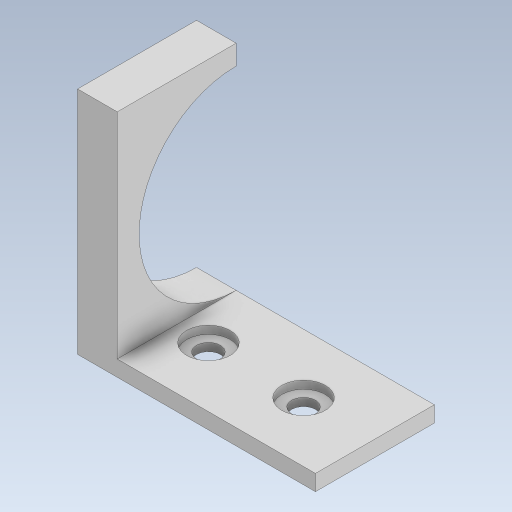
# Autodesk Inventor part: Bracket Motor JGA Kiri
Saved by Autodesk Inventor 2023.5 (Build 275446000, 446)
## iProperties
Created: 2025-09-12
Part Number: Bracket Motor JGA Kiri
Material: Generic
Document SubType Name: Modeling
Designer: Guntur
Density: 1 g/cm^3
Appearance: Default
Author: Guntur
## iProperties of the stored document Bracket Motor JGA Kiri_3DPrint.ipt
Created: 2025-09-14
Part Number: Bracket Motor JGA Kiri_3DPrint
Material: Generic
Document SubType Name: Modeling
Designer: Guntur
Density: 1 g/cm^3
Appearance: Default
Author: Guntur
Autodesk Inventor part; units mm, degrees
ref_plane "YZ Plane" through (0, 0, 0) normal (1, 0, 0) x (0, 1, 0)
ref_plane "XZ Plane" through (0, 0, 0) normal (0, 1, 0) x (-1, 0, 0)
ref_plane "XY Plane" through (0, 0, 0) normal (0, 0, 1) x (1, 0, 0)
sketch "Sketch1" plane through (0, 0, 0) normal (0, 1, 0) x (-1, 0, 0)
  line L0 (15, 7.5) -> (-15, 7.5)
  line L1 (-15, 7.5) -> (-15, -7.5)
  line L2 (-15, -7.5) -> (15, -7.5)
  line L3 (15, -7.5) -> (15, 7.5)
  line L4 (15, 7.5) -> (-15, -7.5) construction
  line L5 (-15, 7.5) -> (15, -7.5) construction
  line L6 (15, 7.5) -> (13, 7.5)
  line L7 (13, 7.5) -> (13, -7.5)
  line L8 (13, -7.5) -> (15, -7.5)
  line L9 (15, -7.5) -> (15, 7.5)
  circle A0 centre (6, 0) radius 1.5
  circle A1 centre (6, 0) radius 2.75
  line L10 (0, 7.5) -> (0, -7.5) construction
  circle A2 centre (-6, 0) radius 1.5
  circle A3 centre (-6, 0) radius 2.75
  point P0 (0, 0)
  dimension "d0" = 30
  dimension "d1" = 15
  dimension "d2" = 2
  dimension "d3" = 3
  dimension "d4" = 5.5
  dimension "d5" = 6
  constraints: 22 end point, 4 centre point, 4 midpoint, 4 parallel, 2 coincident, 2 horizontal, 2 perpendicular, 2 symmetric about line, 1 point on line, 2 other
  measures "d0" distance of L2.end L1.end
  measures "d1" distance of L1.end L0.end
  measures "d2" distance of L8.end L7.end
  measures "d3" diameter of A0
  measures "d4" diameter of A1
  measures "d5" distance of point (0, 0) A0.centre
extrude "Extrusion1" add sketch "Sketch1" along normal blind 2 contours L7 L2 L1 L0
extrude "Extrusion2" add sketch "Sketch1" along normal blind 29 contours L3 L2 L7 L0
extrude "Extrusion3" add sketch "Sketch1" along normal blind 1 contours A1 | A3
sketch "Sketch2" plane through (-13, 2, -7.5) normal (1, 0, 0) x (0, 0, -1)
  line L0 (0, 0) -> (0, 27) projected
  line L1 (0, 0) -> (-15, 0) projected
  circle A0 centre (0, 12.25) radius 12.25
  point P0 (-7.5, -2)
  point P1 (0, 13.5)
  point P2 (0, 24.5)
  dimension "d16" = 24.5
  dimension "d17" = 12.25
  constraints: 1 centre point, 1 midpoint, 1 point on line
  measures "d16" diameter of A0
  measures "d17" distance from line of L1 A0.centre
extrude "Extrusion4" cut sketch "Sketch2" against normal blind 2 contours A0 L0 picked at (-3.685, 9.0749)
sketch "Sketch3" plane through (-13, 2, 7.5) normal (1, 0, 0) x (0, 0, -1)
  line L0 (0, 27) -> (15, 27) projected
  line L1 (15, 27) -> (0, 27)
  line L2 (0, 0) -> (0, 27) projected
  line L3 (0, 27) -> (0, 0)
  line L4 (0, 0) -> (15, 0)
  arc A0 (15, 24.5) -> (15, 0) centre (15, 12.25) ccw projected
  arc A1 (2.75, 12.25) -> (15, 24.5) centre (15, 12.25) ccw
  line L5 (15, 27) -> (15, 24.5)
  line L6 (15, 0) -> (15, 24.5)
  point P0 (7.5, -2)
  constraints: 10 end point, 4 point on circle, 3 collinear, 2 perpendicular, 1 centre point
extrude "Extrusion5" add sketch "Sketch3" along normal blind 3 contours L0 L5 A0 L4 L2
body "Solid1"
